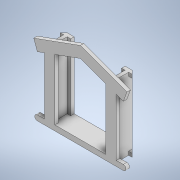
# Autodesk Inventor part: window_test
Saved by Autodesk Inventor 2021 (Build 250183000, 183)
## iProperties
Created: 2021-08-22
Part Number: window_test
Material: Generisch
Document SubType Name: Modeling
Designer: Tilman
Density: 1 g/cm^3
Appearance: Vorgabe
Author: Tilman
Autodesk Inventor part; units mm, degrees
note: some values were not read from the file. Chosen so that the rebuilt part matches the saved one: second side of "Extrusion5".
ref_plane "YZ Plane" through (0, 0, 0) normal (1, 0, 0) x (0, 1, 0)
ref_plane "XZ Plane" through (0, 0, 0) normal (0, 1, 0) x (-1, 0, 0)
ref_plane "XY Plane" through (0, 0, 0) normal (0, 0, 1) x (1, 0, 0)
sketch "Skizze1" plane through (0, 0, 0) normal (0, 0, 1) x (1, 0, 0)
  line L0 (0, 0) -> (18.5, 0)
  line L1 (18.5, 0) -> (18.5, 20.5)
  line L2 (18.5, 20.5) -> (0, 20.5)
  line L3 (0, 20.5) -> (0, 0)
  dimension "d0" = 18.5
  dimension "d1" = 20.5
  constraints: 8 end point, 2 parallel, 1 horizontal, 1 perpendicular
  measures "d0" distance of L1.end L2.end
  measures "d1" distance of L2.end L0.start
extrude "Extrusion1" add sketch "Skizze1" along normal blind 5.5
sketch "Skizze2" plane through (0, 20.5, 0) normal (0, 1, 0) x (1, 0, 0)
  line L0 (18.5, 0) -> (0, 0) projected
  line L1 (0, 0) -> (0, -5.5) projected
  line L2 (18.5, -5.5) -> (0, -5.5) projected
  line L3 (18.5, 0) -> (18.5, -5.5) projected
  line L4 (1, -1) -> (17.5, -1)
  line L5 (17.5, -1) -> (17.5, -4.5)
  line L6 (17.5, -4.5) -> (1, -4.5)
  line L7 (1, -4.5) -> (1, -1)
  line L8 (2, -4.5) -> (2, -5.5)
  line L9 (18.5, -5.5) -> (0, -5.5) projected
  line L10 (16.5, -4.5) -> (16.5, -5.5)
  line L11 (16.5, -1) -> (16.5, 0)
  line L12 (18.5, 0) -> (0, 0) projected
  line L13 (2, -1) -> (2, 0)
  point P0 (1, -2.75)
  point P1 (0, -2.75)
  point P2 (9.25, -1)
  point P3 (9.25, 0)
  point P4 (16.5, -5.5)
  point P5 (2, -5.5)
  point P6 (2, 0)
  point P7 (16.5, 0)
  dimension "d4" = 3.5
  dimension "d5" = 1
  dimension "d8" = 2
  dimension "d9" = 2
  constraints: 16 end point, 12 point on line, 4 midpoint, 3 parallel, 2 perpendicular, 1 horizontal, 1 horizontal alignment, 1 vertical alignment
  measures "d4" distance of L6.end L4.start
  measures "d5" distance between parallel lines of L1 L7
  measures "d8" distance between parallel lines of L1 L8
  measures "d9" distance between parallel lines of L3 L10
extrude "Extrusion2" cut sketch "Skizze2" against normal blind 19 contours L11 L4 L13 L0 | L4 L5 L6 L7 | L2 L8 L6 L10
sketch "Skizze3" plane through (0, 0, 0) normal (0, -1, 0) x (1, 0, 0)
  line L0 (0, 0) -> (18.5, 0) projected
  line L1 (18.5, 0) -> (18.5, 5.5) projected
  line L2 (0, 5.5) -> (18.5, 5.5) projected
  line L3 (0, 0) -> (0, 5.5) projected
  line L4 (0, 0) -> (0, 5.5) projected
  line L5 (0, 1) -> (-1, 1)
  line L6 (-1, 1) -> (0, 0)
  line L7 (18.5, 0) -> (18.5, 5.5) projected
  line L8 (18.5, 1) -> (19.5, 1)
  line L9 (19.5, 1) -> (18.5, 0)
  dimension "d10" = 1
  dimension "d11" = 1
  constraints: 8 end point, 2 equal length, 2 point on line, 1 horizontal, 1 perpendicular
  measures "d10" distance from line of L4.start L5
  measures "d11" distance of L5.start L5.end
extrude "Extrusion3" add sketch "Skizze3" against normal up to surface (20.5 mm away) contours L6 L5 L3 | L1 L8 L9
sketch "Skizze4" plane through (0, 0, 5.5) normal (0, 0, 1) x (1, 0, 0)
  line L0 (16.5, 20.5) -> (16.5, 1.5) projected
  line L1 (16.5, 1.5) -> (2, 1.5) projected
  line L2 (2, 1.5) -> (2, 20.5) projected
  line L3 (2, 20.5) -> (0, 20.5) projected
  line L4 (0, 20.5) -> (0, 0) projected
  line L5 (0, 0) -> (18.5, 0) projected
  line L6 (18.5, 0) -> (18.5, 20.5) projected
  line L7 (18.5, 20.5) -> (16.5, 20.5) projected
  line L8 (0, 20.5) -> (0, 0) projected
  line L9 (-1, 0) -> (-1, 20.5) projected
  line L10 (0, 19.5) -> (-1, 19.5)
  line L11 (-1, 19.5) -> (-1, 1)
  line L12 (-1, 1) -> (0, 1)
  line L13 (0, 1) -> (0, 19.5)
  line L14 (18.5, 0) -> (18.5, 20.5) projected
  line L15 (19.5, 0) -> (19.5, 20.5) projected
  line L16 (18.5, 19.5) -> (19.5, 19.5)
  line L17 (19.5, 19.5) -> (19.5, 1)
  line L18 (19.5, 1) -> (18.5, 1)
  line L19 (18.5, 1) -> (18.5, 19.5)
  line L20 (0, 20.5) -> (-1, 20.5) projected
  point P0 (0, 10.25)
  point P1 (18.5, 10.25)
  dimension "d14" = 1
  constraints: 16 end point, 5 parallel, 4 midpoint, 4 point on line, 2 horizontal, 2 perpendicular
  measures "d14" distance between parallel lines of L10 L20
extrude "Extrusion4" cut sketch "Skizze4" against normal through all contours L16 L15 L18 L6 | L4 L12 L9 L10
sketch "Skizze5" plane through (0, 0, 5.5) normal (0, 0, 1) x (1, 0, 0)
  line L0 (16.5, 20.5) -> (16.5, 1.5) projected
  line L1 (16.5, 1.5) -> (2, 1.5) projected
  line L2 (2, 1.5) -> (2, 20.5) projected
  line L3 (2, 20.5) -> (0, 20.5) projected
  line L4 (0, 20.5) -> (0, 0) projected
  line L5 (0, 0) -> (18.5, 0) projected
  line L6 (18.5, 0) -> (18.5, 20.5) projected
  line L7 (18.5, 20.5) -> (16.5, 20.5) projected
  line L8 (-3, 1.5) -> (21.5, 1.5)
  line L9 (21.5, 0) -> (-3, 0)
  arc A0 (-3, 1.5) -> (-3, 0) centre (-3, 0.75) ccw
  arc A1 (21.5, 0) -> (21.5, 1.5) centre (21.5, 0.75) ccw
  line L10 (-3, 17.0839) -> (-4.0261, 19.903)
  line L11 (-4.0261, 19.903) -> (9.25, 24.7351)
  line L12 (9.25, 24.7351) -> (22.5261, 19.903)
  line L13 (22.5261, 19.903) -> (21.5, 17.0839)
  line L14 (21.5, 17.0839) -> (9.25, 21.5425)
  line L15 (9.25, 21.5425) -> (-3, 17.0839)
  line L16 (16.5, 1.5) -> (2, 1.5) projected
  line L17 (-1, 17.8118) -> (-1, 1.5)
  line L18 (19.5, 1.5) -> (19.5, 17.8118)
  line L19 (2.513, 19.0905) -> (1.487, 21.9095) construction
  point P0 (9.25, 1.5)
  point P1 (18.5, 1.5)
  point P2 (0, 1.5)
  point P3 (9.25, 1.5)
  point P4 (2, 18.9037)
  point P5 (16.5, 18.9037)
  dimension "d18" = 3
  dimension "d31" = 20
  dimension "d32" = 3
  dimension "d33" = 1
  constraints: 22 end point, 8 point on line, 4 equal length, 4 midpoint, 4 point on circle, 4 tangent, 3 perpendicular, 3 vertical alignment, 2 centre point, 2 parallel, 2 vertical, 1 horizontal
  measures "d18" distance from line of L4 A0.centre
  measures "d31" angle of L1 L15
  measures "d32" distance of L10.start L10.end
  measures "d33" distance between parallel lines of L4 L17
extrude "Extrusion5" add sketch "Skizze5" against normal blind 1 contours L0 L14 L15 L2 L3 L4 L10 L11 L12 L13 L6 L7 | L8 L6 L5 L4 L1 | L14 L18 L8 L6 | L8 A1 L9 L6 | L8 L17 L15 L4 | L4 L9 A0 L8
equation "\"d9\" = d8"
